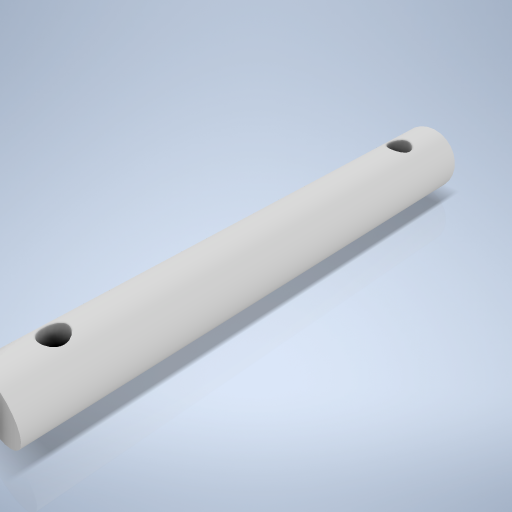
# Autodesk Inventor part: 21
Saved by Autodesk Inventor 2024.2 (Build 282272000, 272)
## iProperties
Created: 2024-05-05
Part Number: 21
Material: Generisch
Document SubType Name: Modeling
Designer: Fabri
Density: 1 g/cm^3
Appearance: Vorgabe
Author: Fabri
Autodesk Inventor part; units mm, degrees
ref_plane "YZ Plane" through (0, 0, 0) normal (1, 0, 0) x (0, 1, 0)
ref_plane "XZ Plane" through (0, 0, 0) normal (0, 1, 0) x (-1, 0, 0)
sketch "Skizze1" plane through (0, 0, 0) normal (0, 1, 0) x (-1, 0, 0)
  circle A0 centre (0, 0) radius 8
  dimension "d0" = 16
  constraints: 1 centre point, 1 coincident
  measures "d0" diameter of A0
extrude "Extrusion1" add sketch "Skizze1" along normal blind 120
ref_plane "Arbeitsebene1" through (0, 0, 8) normal (0, 0, 1) x (1, 0, 0)
sketch "Skizze2" plane through (0, 0, 8) normal (0, 0, 1) x (1, 0, 0)
  line L0 (8, 120) -> (-8, 120) projected
  line L1 (8, 0) -> (-8, 0) projected
  line L2 (-8, 0) -> (-8, 120) projected
  line L3 (-8, 60) -> (7.5453, 60)
  point P0 (0, 0)
  point P1 (0, 12.75)
  point P2 (0, 107.25)
  dimension "d13" = 94.5
  dimension "d14" = 120
  constraints: 2 end point, 2 vertical alignment, 1 horizontal, 1 midpoint, 1 symmetric about line
  measures "d13" distance of point (0, 107.25) point (0, 12.75)
  measures "d14" distance between parallel lines of L0 L1
hole "Bohrung1" at (0, 12.75, 8) at (0, 107.25, 8) direction (0, 0, -1) diameter 6 end through all
